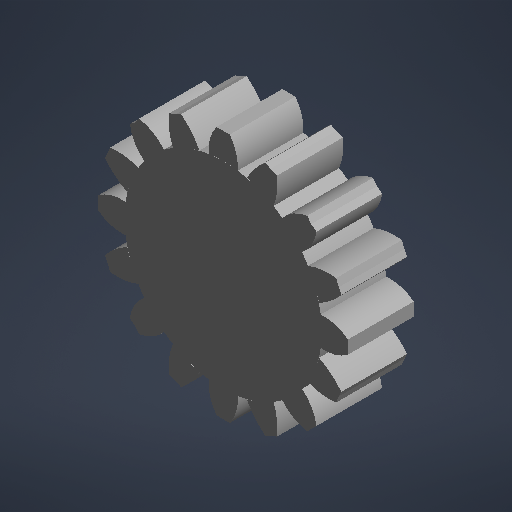
# Autodesk Inventor part: test_gear_cad_model
Saved by Autodesk Inventor 2026 (Build 300175050, 175E)
## iProperties
Part Number: test_gear_cad_model
Material: Generic
Document SubType Name: Modeling
Designer: Administrator
Appearance: Default
Author: Administrator
Autodesk Inventor part; units mm, degrees
ref_plane "YZ Plane" through (0, 0, 0) normal (1, 0, 0) x (0, 1, 0)
ref_plane "XZ Plane" through (0, 0, 0) normal (0, 1, 0) x (-1, 0, 0)
ref_plane "Work Plane1" through (0, 0, 0) normal (0, 0, 1) x (1, 0, 0)
sketch "Sketch1" plane through (0, 0, 0) normal (0, 0, 1) x (1, 0, 0)
  circle A0 centre (0, 0) radius 0.075
  arc A1 (-0.011, -0.074) -> (0.011, -0.074) centre (0, -0.014) ccw
  arc A2 (-0.011, -0.074) -> (-0.005, -0.095) centre (0.0188, -0.0768) ccw
  line L0 (0, -0.095) -> (-0.005, -0.095)
  line L1 (0.005, -0.095) -> (0, -0.095)
  arc A3 (0.005, -0.095) -> (0.011, -0.074) centre (-0.0188, -0.0768) ccw
  arc A4 (0.018, -0.073) -> (0.038, -0.064) centre (-0.0002, -0.0059) ccw
  arc A5 (0.018, -0.073) -> (0.032, -0.09) centre (0.0675, -0.0465) ccw
  line L2 (0.036, -0.088) -> (0.032, -0.09)
  line L3 (0.041, -0.086) -> (0.036, -0.088)
  arc A6 (0.041, -0.086) -> (0.038, -0.064) centre (-0.0008, -0.0805) ccw
  arc A7 (0.064, -0.038) -> (0.073, -0.018) centre (0.0059, 0.0002) ccw
  arc A8 (0.064, -0.038) -> (0.086, -0.041) centre (0.0805, 0.0008) ccw
  line L4 (0.088, -0.036) -> (0.086, -0.041)
  line L5 (0.09, -0.032) -> (0.088, -0.036)
  arc A9 (0.09, -0.032) -> (0.073, -0.018) centre (0.0465, -0.0675) ccw
  arc A10 (0.074, -0.011) -> (0.074, 0.011) centre (0.014, 0) ccw
  arc A11 (0.074, -0.011) -> (0.095, -0.005) centre (0.0768, 0.0188) ccw
  line L6 (0.095, 0) -> (0.095, -0.005)
  line L7 (0.095, 0.005) -> (0.095, 0)
  arc A12 (0.095, 0.005) -> (0.074, 0.011) centre (0.0768, -0.0188) ccw
  arc A13 (0.045, -0.06) -> (0.06, -0.045) centre (-0.0035, 0.0035) ccw
  arc A14 (0.045, -0.06) -> (0.064, -0.071) centre (0.0687, -0.041) ccw
  line L8 (0.067, -0.067) -> (0.064, -0.071)
  line L9 (0.071, -0.064) -> (0.067, -0.067)
  arc A15 (0.071, -0.064) -> (0.06, -0.045) centre (0.041, -0.0687) ccw
  arc A16 (0.073, 0.018) -> (0.064, 0.038) centre (0.0059, -0.0002) ccw
  arc A17 (0.073, 0.018) -> (0.09, 0.032) centre (0.0465, 0.0675) ccw
  line L10 (0.088, 0.036) -> (0.09, 0.032)
  line L11 (0.086, 0.041) -> (0.088, 0.036)
  arc A18 (0.086, 0.041) -> (0.064, 0.038) centre (0.0805, -0.0008) ccw
  arc A19 (0.06, 0.045) -> (0.045, 0.06) centre (-0.0035, -0.0035) ccw
  arc A20 (0.06, 0.045) -> (0.071, 0.064) centre (0.041, 0.0687) ccw
  line L12 (0.067, 0.067) -> (0.071, 0.064)
  line L13 (0.064, 0.071) -> (0.067, 0.067)
  arc A21 (0.064, 0.071) -> (0.045, 0.06) centre (0.0687, 0.041) ccw
  arc A22 (0.038, 0.064) -> (0.018, 0.073) centre (-0.0002, 0.0059) ccw
  arc A23 (0.038, 0.064) -> (0.041, 0.086) centre (-0.0008, 0.0805) ccw
  line L14 (0.036, 0.088) -> (0.041, 0.086)
  line L15 (0.032, 0.09) -> (0.036, 0.088)
  arc A24 (0.032, 0.09) -> (0.018, 0.073) centre (0.0675, 0.0465) ccw
  arc A25 (-0.038, -0.064) -> (-0.018, -0.073) centre (0.0002, -0.0059) ccw
  arc A26 (-0.038, -0.064) -> (-0.041, -0.086) centre (0.0008, -0.0805) ccw
  line L16 (-0.036, -0.088) -> (-0.041, -0.086)
  line L17 (-0.032, -0.09) -> (-0.036, -0.088)
  arc A27 (-0.032, -0.09) -> (-0.018, -0.073) centre (-0.0675, -0.0465) ccw
  arc A28 (-0.06, -0.045) -> (-0.045, -0.06) centre (0.0035, 0.0035) ccw
  arc A29 (-0.06, -0.045) -> (-0.071, -0.064) centre (-0.041, -0.0687) ccw
  line L18 (-0.067, -0.067) -> (-0.071, -0.064)
  line L19 (-0.064, -0.071) -> (-0.067, -0.067)
  arc A30 (-0.064, -0.071) -> (-0.045, -0.06) centre (-0.0687, -0.041) ccw
  arc A31 (-0.073, -0.018) -> (-0.064, -0.038) centre (-0.0059, 0.0002) ccw
  arc A32 (-0.073, -0.018) -> (-0.09, -0.032) centre (-0.0465, -0.0675) ccw
  line L20 (-0.088, -0.036) -> (-0.09, -0.032)
  line L21 (-0.086, -0.041) -> (-0.088, -0.036)
  arc A33 (-0.086, -0.041) -> (-0.064, -0.038) centre (-0.0805, 0.0008) ccw
  arc A34 (-0.074, 0.011) -> (-0.074, -0.011) centre (-0.014, 0) ccw
  arc A35 (-0.074, 0.011) -> (-0.095, 0.005) centre (-0.0768, -0.0188) ccw
  line L22 (-0.095, 0) -> (-0.095, 0.005)
  line L23 (-0.095, -0.005) -> (-0.095, 0)
  arc A36 (-0.095, -0.005) -> (-0.074, -0.011) centre (-0.0768, 0.0188) ccw
  arc A37 (-0.064, 0.038) -> (-0.073, 0.018) centre (-0.0059, -0.0002) ccw
  arc A38 (-0.064, 0.038) -> (-0.086, 0.041) centre (-0.0805, -0.0008) ccw
  line L24 (-0.088, 0.036) -> (-0.086, 0.041)
  line L25 (-0.09, 0.032) -> (-0.088, 0.036)
  arc A39 (-0.09, 0.032) -> (-0.073, 0.018) centre (-0.0465, 0.0675) ccw
  arc A40 (-0.045, 0.06) -> (-0.06, 0.045) centre (0.0035, -0.0035) ccw
  arc A41 (-0.045, 0.06) -> (-0.064, 0.071) centre (-0.0687, 0.041) ccw
  line L26 (-0.067, 0.067) -> (-0.064, 0.071)
  line L27 (-0.071, 0.064) -> (-0.067, 0.067)
  arc A42 (-0.071, 0.064) -> (-0.06, 0.045) centre (-0.041, 0.0687) ccw
  arc A43 (-0.018, 0.073) -> (-0.038, 0.064) centre (0.0002, 0.0059) ccw
  arc A44 (-0.018, 0.073) -> (-0.032, 0.09) centre (-0.0675, 0.0465) ccw
  line L28 (-0.036, 0.088) -> (-0.032, 0.09)
  line L29 (-0.041, 0.086) -> (-0.036, 0.088)
  arc A45 (-0.041, 0.086) -> (-0.038, 0.064) centre (0.0008, 0.0805) ccw
  arc A46 (0, 0.075) -> (-0.011, 0.074) centre (-0.0025, 0.0415) ccw
  arc A47 (-0.005, 0.095) -> (-0.011, 0.074) centre (0.0188, 0.0768) ccw
  line L30 (0, 0.095) -> (-0.005, 0.095)
  line L31 (0, 0.075) -> (0, 0.095)
  arc A48 (0.011, 0.074) -> (0, 0.075) centre (0.0025, 0.0415) ccw
  arc A49 (0.011, 0.074) -> (0.005, 0.095) centre (-0.0188, 0.0768) ccw
  line L32 (0, 0.095) -> (0.005, 0.095)
  line L33 (0, 0.075) -> (0, 0.095)
  constraints: 98 point on circle, 68 end point, 50 centre point
extrude "Extrusion1" add sketch "Sketch1" along normal blind 0.05
body "Solid1"
